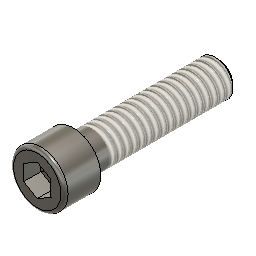
IntakePrototype (Autodesk Fusion 360 archive; units mm, degrees)
design "Hexagon Socket Head Cap Screw ANSI B18.3 - 1/4-20 UNC x 1 Steel Grade 2 Plain"
description: Hexagon Socket Head Cap Screw ANSI B18.3 - 1/4-20 UNC x 1
Autodesk Fusion 360 part; units mm, degrees
sketch "Sketch1" plane through (0, 0, 0) normal (0, 1, 0) x (1, 0, 0)
  line L0 (-3.175, 0) -> (-3.175, 25.4)
  line L1 (-3.175, 25.4) -> (0, 25.4)
  line L2 (0, 25.4) -> (0, -6.35)
  line L3 (-3.175, 0) -> (-4.7625, 0)
  line L4 (-4.7625, 0) -> (-4.7625, -6.35)
  line L5 (-4.7625, -6.35) -> (0, -6.35)
  dimension "d9" = 6.35
  dimension "d66" = 9.525
  dimension "d68" = 25.4
  dimension "d79" = 6.35
  constraint perpendicular L0 L1
  constraint collinear origin L1.end L2.end
  constraint perpendicular L0 L3
  constraint coincident origin L3
  constraint vertical L0
  constraint vertical L2
  constraint parallel L2 L4
  constraint coincident L2 L5.end
  constraint perpendicular L2 L5
  measures "d68" distance of origin L1.end
  measures "d79" distance of L3.end L4.end
revolve "Revolve1" add sketch "Sketch1" angle 360 about axis through (0, 0, -25.4) along (0, 0, 1)
ref_plane "WorkPlane1" through (0, 0, 6.35) normal (0, 0, 1) x (1, 0, 0)
sketch "Sketch6" plane through (0, 0, 6.35) normal (0, 0, 1) x (1, 0, 0)
  line L0 (-2.3876, 0) -> (2.3876, 0) construction
  line L1 (0, 0) -> (-2.3876, 1.3785)
  line L2 (-2.3876, -1.3785) -> (-2.3876, 1.3785)
  line L3 (-2.3876, -1.3785) -> (0, 0)
  dimension "d72" = 4.7752
  dimension "d106" = 150
  constraint horizontal L0
  constraint midpoint L1.start L0
  constraint coincident L1.start L3.end
  constraint perpendicular L0 L2
  constraint midpoint L0.start L2
  constraint coincident L1.end L2.end
  measures "d72" distance of L0.start L0.end
  measures "d106" angle of L0 L1
extrude "Extrude1" cut sketch "Sketch6" against normal blind 3.048
pattern_circular "C-Pattern1" count 6 over 360 about axis through (0, 0, 1.75) along (0, 0, 1) of "Extrude1"
extrude "Extrude2" cut 1 faces at (0, 0, 3.302) along direction (0, 0, -1) blind 3.048 draft -85
thread "Thread2" "ANSI Unified Screw Threads 0.25 1/4-20 UNC 2A" major diameter 6.2205 minor diameter 4.8108 pitch 1.27 angle 60 resizes the face on face at (-3.1711, 0.1583, -16.9333) from (0, 0, -3.1752) to (0, 0, -25.4)
fillet "Fillet4" radius 0.635 1 edges at (-4.4402, 1.7222, 6.35)
sketch "Sketch7" plane through (0, 0, 0) normal (0, 1, 0) x (1, 0, 0)
  line L0 (-3.2385, 25.4) -> (-3.2385, 24.6444)
  line L1 (-3.2385, 24.6444) -> (-2.4193, 25.4)
  line L2 (0, 25.4) -> (0, -6.35)
  line L3 (-3.2385, 25.4) -> (0, 25.4)
  dimension "d103" = 3.2385
  dimension "d104" = 0.7556
  dimension "d105" = 2.4194
  constraint coincident L2.start L3.end
  constraint perpendicular L2 L3
  constraint coincident L1.end L3
  constraint perpendicular L0 L3
  measures "d103" distance of origin L0
  measures "d104" vertical distance of L0.end L1.end
  measures "d105" horizontal distance of origin L1.end
revolve "Revolve3" cut sketch "Sketch7" angle 360 about axis through (0, 0, 1.75) along (0, 0, 1)
equation "d9 = adsk_nomdia"
equation "d31 = -adsk_keyend"
equation "d66 = adsk_headdia"
equation "d68 = adsk_nomlen"
equation "d71 = adsk_headh"
equation "d72 = adsk_waflat"
equation "d76 = -adsk_keyend"
equation "d79 = adsk_headh"
equation "adsk_nomlen = 1.00 in"
equation "adsk_headh = 0.25 in"
equation "adsk_headdia = 0.375 in"
equation "adsk_nomdia = 0.25 in"
equation "adsk_waflat = 0.188 in"
equation "adsk_keyend = 0.12 in"
equation "adsk_thrlen = 0.8749921 in"
equation "d93 = adsk_nomdia * 0.1"
equation "adsk_startlen = 0.02975 in"
equation "adsk_endpointdia = 0.1905 in"
equation "d103 = adsk_nomdia * 0.51"
equation "d104 = adsk_startlen"
equation "d105 = adsk_endpointdia / 2"
